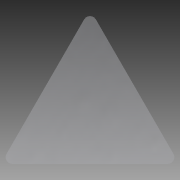
# Autodesk Inventor part: g16-pixel
Saved by Autodesk Inventor 2013 (Build 170138000, 138)
## iProperties
Created: 2013-03-21
Part Number: g16-pixel
Material: Acrylic, Clear
Document SubType Name: Modeling
Designer: TechShop Member
Density: 1 g/cm^3
Author: TechShop Member
Autodesk Inventor part; units mm, degrees
ref_plane "YZ Plane" through (0, 0, 0) normal (1, 0, 0) x (0, 1, 0)
ref_plane "XZ Plane" through (0, 0, 0) normal (0, 1, 0) x (-1, 0, 0)
ref_plane "XY Plane" through (0, 0, 0) normal (0, 0, 1) x (1, 0, 0)
sketch "Sketch1" plane through (0, 0, 0) normal (0, 1, 0) x (-1, 0, 0)
  line L0 (33.333, 0) -> (0, 0) construction
  line L1 (0, 0) -> (16.6665, 28.8672) construction
  line L2 (16.6665, 28.8672) -> (33.333, 0) construction
  line L3 (32.467, 0.5) -> (0.866, 0.5) construction
  line L4 (0.866, 0.5) -> (16.6665, 27.8672) construction
  line L5 (16.6665, 27.8672) -> (32.467, 0.5) construction
  line L6 (16.6665, 0.5) -> (16.6665, 0) construction
  line L7 (8.7663, 14.1836) -> (8.3333, 14.4336) construction
  line L8 (24.5667, 14.1836) -> (24.9998, 14.4336) construction
  arc A0 (1.9053, 2.3) -> (2.9445, 0.5) centre (2.9445, 1.7) ccw projected
  arc A1 (17.7057, 26.0672) -> (15.6273, 26.0672) centre (16.6665, 25.4672) ccw projected
  arc A2 (30.3885, 0.5) -> (31.4277, 2.3) centre (30.3885, 1.7) ccw projected
  line L9 (30.3885, 0.5) -> (2.9445, 0.5) projected
  line L10 (1.9053, 2.3) -> (15.6273, 26.0672) projected
  line L11 (17.7057, 26.0672) -> (31.4277, 2.3) projected
  circle A3 centre (31.7742, 0.9) radius 0.4 construction
  line L12 (31.4277, 1.1) -> (32.1206, 0.7) construction
  circle A4 centre (33.333, 0) radius 3 construction
  line L13 (16.6665, 0) -> (16.6665, -0.5) construction
  line L14 (31.4277, 1.1) -> (30.7349, 1.5) construction
  point P0 (0, 0)
  constraints: 1 other
extrude "Extrusion1" add sketch "Sketch1" along normal blind 2.75
sketch "Triangle Hole Template" plane through (0, 0, 0) normal (0, 0, 1) x (1, 0, 0)
  line L0 (-99.9974, -57.7156) -> (-66.6644, -57.7156) construction
  line L1 (-66.6644, -57.7156) -> (-83.3309, -86.5829) construction
  line L2 (-83.3309, -86.5829) -> (-99.9974, -57.7156) construction
  line L3 (-99.1314, -58.2156) -> (-67.5304, -58.2156) construction
  line L4 (-67.5304, -58.2156) -> (-83.3309, -85.5829) construction
  line L5 (-83.3309, -85.5829) -> (-99.1314, -58.2156) construction
  line L6 (-83.3309, -58.2156) -> (-83.3309, -57.7156) construction
  line L7 (-75.4307, -71.8992) -> (-74.9976, -72.1492) construction
  line L8 (-91.2311, -71.8992) -> (-91.6641, -72.1492) construction
  arc A0 (-68.5696, -60.0156) -> (-69.6089, -58.2156) centre (-69.6089, -59.4156) ccw
  arc A1 (-84.3701, -83.7829) -> (-82.2917, -83.7829) centre (-83.3309, -83.1829) ccw
  arc A2 (-97.0529, -58.2156) -> (-98.0921, -60.0156) centre (-97.0529, -59.4156) ccw
  line L9 (-97.0529, -58.2156) -> (-69.6089, -58.2156)
  line L10 (-68.5696, -60.0156) -> (-82.2917, -83.7829)
  line L11 (-84.3701, -83.7829) -> (-98.0921, -60.0156)
  circle A3 centre (-98.4385, -58.6156) radius 0.4 construction
  line L12 (-98.0921, -58.8156) -> (-98.785, -58.4156) construction
  circle A4 centre (-99.9974, -57.7156) radius 3 construction
  line L13 (-83.3309, -57.7156) -> (-83.3309, -57.2156) construction
  line L14 (-98.0921, -58.8156) -> (-97.3993, -59.2156) construction
  point P0 (-85.6081, -66.0431)
  dimension "d24" = 6
  dimension "Pixel_BorderWidth" = 1
  dimension "Pixel_Stride" = 33.333
  measures "Pixel_BorderWidth" distance of L13.end L6.start
  measures "Pixel_Stride" distance of L0.start L0.end
sketch "Triangle Hole Template x16" plane through (0, 0, 0) normal (0, 0, 1) x (1, 0, 0)
  line L0 (-16.6681, -28.8484) -> (-50.0011, -28.8484) construction
  line L1 (-50.0011, -28.8484) -> (-33.3346, 0.0188) construction
  line L2 (-33.3346, 0.0188) -> (-16.6681, -28.8484) construction
  line L3 (-17.5341, -28.3484) -> (-49.1351, -28.3484) construction
  line L4 (-49.1351, -28.3484) -> (-33.3346, -0.9812) construction
  line L5 (-33.3346, -0.9812) -> (-17.5341, -28.3484) construction
  line L6 (-33.3346, -28.3484) -> (-33.3346, -28.8484) construction
  line L7 (-41.2348, -14.6648) -> (-41.6679, -14.4148) construction
  line L8 (-25.4344, -14.6648) -> (-25.0014, -14.4148) construction
  arc A0 (-48.0959, -26.5484) -> (-47.0566, -28.3484) centre (-47.0566, -27.1484) ccw
  arc A1 (-32.2954, -2.7812) -> (-34.3738, -2.7812) centre (-33.3346, -3.3812) ccw
  arc A2 (-19.6126, -28.3484) -> (-18.5734, -26.5484) centre (-19.6126, -27.1484) ccw
  line L9 (-19.6126, -28.3484) -> (-47.0566, -28.3484)
  line L10 (-48.0959, -26.5484) -> (-34.3738, -2.7812)
  line L11 (-32.2954, -2.7812) -> (-18.5734, -26.5484)
  circle A3 centre (-18.227, -27.9484) radius 0.4 construction
  line L12 (-18.5734, -27.7484) -> (-17.8805, -28.1484) construction
  circle A4 centre (-16.6681, -28.8484) radius 3 construction
  line L13 (-33.3346, -28.8484) -> (-33.3346, -29.3484) construction
  line L14 (-18.5734, -27.7484) -> (-19.2662, -27.3484) construction
  line L15 (-49.9979, -28.8484) -> (-16.6649, -28.8484) construction
  line L16 (-16.6649, -28.8484) -> (-33.3314, -57.7156) construction
  line L17 (-33.3314, -57.7156) -> (-49.9979, -28.8484) construction
  line L18 (-49.1319, -29.3484) -> (-17.5309, -29.3484) construction
  line L19 (-17.5309, -29.3484) -> (-33.3314, -56.7156) construction
  line L20 (-33.3314, -56.7156) -> (-49.1319, -29.3484) construction
  line L21 (-33.3314, -29.3484) -> (-33.3314, -28.8484) construction
  line L22 (-25.4312, -43.032) -> (-24.9981, -43.282) construction
  line L23 (-41.2316, -43.032) -> (-41.6646, -43.282) construction
  arc A5 (-18.5701, -31.1484) -> (-19.6094, -29.3484) centre (-19.6094, -30.5484) ccw
  arc A6 (-34.3706, -54.9156) -> (-32.2922, -54.9156) centre (-33.3314, -54.3156) ccw
  arc A7 (-47.0534, -29.3484) -> (-48.0926, -31.1484) centre (-47.0534, -30.5484) ccw
  line L24 (-47.0534, -29.3484) -> (-19.6094, -29.3484)
  line L25 (-18.5701, -31.1484) -> (-32.2922, -54.9156)
  line L26 (-34.3706, -54.9156) -> (-48.0926, -31.1484)
  circle A8 centre (-48.439, -29.7484) radius 0.4 construction
  line L27 (-48.0926, -29.9484) -> (-48.7855, -29.5484) construction
  circle A9 centre (-49.9979, -28.8484) radius 3 construction
  line L28 (-33.3314, -28.8484) -> (-33.3314, -28.3484) construction
  line L29 (-48.0926, -29.9484) -> (-47.3998, -30.3484) construction
  line L30 (-66.6676, 0.0188) -> (-33.3346, 0.0188) construction
  line L31 (-33.3346, 0.0188) -> (-50.0011, -28.8484) construction
  line L32 (-50.0011, -28.8484) -> (-66.6676, 0.0188) construction
  line L33 (-65.8016, -0.4812) -> (-34.2006, -0.4812) construction
  line L34 (-34.2006, -0.4812) -> (-50.0011, -27.8484) construction
  line L35 (-50.0011, -27.8484) -> (-65.8016, -0.4812) construction
  line L36 (-50.0011, -0.4812) -> (-50.0011, 0.0188) construction
  line L37 (-42.1009, -14.1648) -> (-41.6679, -14.4148) construction
  line L38 (-57.9013, -14.1648) -> (-58.3344, -14.4148) construction
  arc A10 (-35.2399, -2.2812) -> (-36.2791, -0.4812) centre (-36.2791, -1.6812) ccw
  arc A11 (-51.0403, -26.0484) -> (-48.9619, -26.0484) centre (-50.0011, -25.4484) ccw
  arc A12 (-63.7231, -0.4812) -> (-64.7624, -2.2812) centre (-63.7231, -1.6812) ccw
  line L39 (-63.7231, -0.4812) -> (-36.2791, -0.4812)
  line L40 (-35.2399, -2.2812) -> (-48.9619, -26.0484)
  line L41 (-51.0403, -26.0484) -> (-64.7624, -2.2812)
  circle A13 centre (-65.1088, -0.8812) radius 0.4 construction
  line L42 (-64.7624, -1.0812) -> (-65.4552, -0.6812) construction
  circle A14 centre (-66.6676, 0.0188) radius 3 construction
  line L43 (-50.0011, 0.0188) -> (-50.0011, 0.5188) construction
  line L44 (-64.7624, -1.0812) -> (-64.0695, -1.4812) construction
  line L45 (-33.3314, 0.0188) -> (0.0016, 0.0188) construction
  line L46 (0.0016, 0.0188) -> (-16.6649, -28.8484) construction
  line L47 (-16.6649, -28.8484) -> (-33.3314, 0.0188) construction
  line L48 (-32.4654, -0.4812) -> (-0.8644, -0.4812) construction
  line L49 (-0.8644, -0.4812) -> (-16.6649, -27.8484) construction
  line L50 (-16.6649, -27.8484) -> (-32.4654, -0.4812) construction
  line L51 (-16.6649, -0.4812) -> (-16.6649, 0.0188) construction
  line L52 (-8.7647, -14.1648) -> (-8.3316, -14.4148) construction
  line L53 (-24.5651, -14.1648) -> (-24.9981, -14.4148) construction
  arc A15 (-1.9036, -2.2812) -> (-2.9429, -0.4812) centre (-2.9429, -1.6812) ccw
  arc A16 (-17.7041, -26.0484) -> (-15.6257, -26.0484) centre (-16.6649, -25.4484) ccw
  arc A17 (-30.3869, -0.4812) -> (-31.4261, -2.2812) centre (-30.3869, -1.6812) ccw
  line L54 (-30.3869, -0.4812) -> (-2.9429, -0.4812)
  line L55 (-1.9036, -2.2812) -> (-15.6257, -26.0484)
  line L56 (-17.7041, -26.0484) -> (-31.4261, -2.2812)
  circle A18 centre (-31.7725, -0.8812) radius 0.4 construction
  line L57 (-31.4261, -1.0812) -> (-32.119, -0.6812) construction
  circle A19 centre (-33.3314, 0.0188) radius 3 construction
  line L58 (-16.6649, 0.0188) -> (-16.6649, 0.5188) construction
  line L59 (-31.4261, -1.0812) -> (-30.7333, -1.4812) construction
  line L60 (-83.317, -28.8188) -> (-49.984, -28.8188) construction
  line L61 (-49.984, -28.8188) -> (-66.6505, -57.686) construction
  line L62 (-66.6505, -57.686) -> (-83.317, -28.8188) construction
  line L63 (-82.451, -29.3188) -> (-50.85, -29.3188) construction
  line L64 (-50.85, -29.3188) -> (-66.6505, -56.686) construction
  line L65 (-66.6505, -56.686) -> (-82.451, -29.3188) construction
  line L66 (-66.6505, -29.3188) -> (-66.6505, -28.8188) construction
  line L67 (-58.7503, -43.0024) -> (-58.3173, -43.2524) construction
  line L68 (-74.5507, -43.0024) -> (-74.9838, -43.2524) construction
  arc A20 (-51.8893, -31.1188) -> (-52.9285, -29.3188) centre (-52.9285, -30.5188) ccw
  arc A21 (-67.6897, -54.886) -> (-65.6113, -54.886) centre (-66.6505, -54.286) ccw
  arc A22 (-80.3725, -29.3188) -> (-81.4117, -31.1188) centre (-80.3725, -30.5188) ccw
  line L69 (-80.3725, -29.3188) -> (-52.9285, -29.3188)
  line L70 (-51.8893, -31.1188) -> (-65.6113, -54.886)
  line L71 (-67.6897, -54.886) -> (-81.4117, -31.1188)
  circle A23 centre (-81.7582, -29.7188) radius 0.4 construction
  line L72 (-81.4117, -29.9188) -> (-82.1046, -29.5188) construction
  circle A24 centre (-83.317, -28.8188) radius 3 construction
  line L73 (-66.6505, -28.8188) -> (-66.6505, -28.3188) construction
  line L74 (-81.4117, -29.9188) -> (-80.7189, -30.3188) construction
  line L75 (-99.9974, 0.0188) -> (-66.6644, 0.0188) construction
  line L76 (-66.6644, 0.0188) -> (-83.3309, -28.8484) construction
  line L77 (-83.3309, -28.8484) -> (-99.9974, 0.0188) construction
  line L78 (-99.1314, -0.4812) -> (-67.5304, -0.4812) construction
  line L79 (-67.5304, -0.4812) -> (-83.3309, -27.8484) construction
  line L80 (-83.3309, -27.8484) -> (-99.1314, -0.4812) construction
  line L81 (-83.3309, -0.4812) -> (-83.3309, 0.0188) construction
  line L82 (-75.4307, -14.1648) -> (-74.9976, -14.4148) construction
  line L83 (-91.2311, -14.1648) -> (-91.6641, -14.4148) construction
  arc A25 (-68.5696, -2.2812) -> (-69.6089, -0.4812) centre (-69.6089, -1.6812) ccw
  arc A26 (-84.3701, -26.0484) -> (-82.2917, -26.0484) centre (-83.3309, -25.4484) ccw
  arc A27 (-97.0529, -0.4812) -> (-98.0921, -2.2812) centre (-97.0529, -1.6812) ccw
  line L84 (-97.0529, -0.4812) -> (-69.6089, -0.4812)
  line L85 (-68.5696, -2.2812) -> (-82.2917, -26.0484)
  line L86 (-84.3701, -26.0484) -> (-98.0921, -2.2812)
  circle A28 centre (-98.4385, -0.8812) radius 0.4 construction
  line L87 (-98.0921, -1.0812) -> (-98.785, -0.6812) construction
  circle A29 centre (-99.9974, 0.0188) radius 3 construction
  line L88 (-83.3309, 0.0188) -> (-83.3309, 0.5188) construction
  line L89 (-98.0921, -1.0812) -> (-97.3993, -1.4812) construction
  line L90 (-133.3304, -0.008) -> (-99.9974, -0.008) construction
  line L91 (-99.9974, -0.008) -> (-116.6639, -28.8752) construction
  line L92 (-116.6639, -28.8752) -> (-133.3304, -0.008) construction
  line L93 (-132.4644, -0.508) -> (-100.8634, -0.508) construction
  line L94 (-100.8634, -0.508) -> (-116.6639, -27.8752) construction
  line L95 (-116.6639, -27.8752) -> (-132.4644, -0.508) construction
  line L96 (-116.6639, -0.508) -> (-116.6639, -0.008) construction
  line L97 (-108.7637, -14.1916) -> (-108.3306, -14.4416) construction
  line L98 (-124.5641, -14.1916) -> (-124.9971, -14.4416) construction
  arc A30 (-101.9026, -2.308) -> (-102.9419, -0.508) centre (-102.9419, -1.708) ccw
  arc A31 (-117.7031, -26.0752) -> (-115.6247, -26.0752) centre (-116.6639, -25.4752) ccw
  arc A32 (-130.3859, -0.508) -> (-131.4251, -2.308) centre (-130.3859, -1.708) ccw
  line L99 (-130.3859, -0.508) -> (-102.9419, -0.508)
  line L100 (-101.9026, -2.308) -> (-115.6247, -26.0752)
  line L101 (-117.7031, -26.0752) -> (-131.4251, -2.308)
  circle A33 centre (-131.7715, -0.908) radius 0.4 construction
  line L102 (-131.4251, -1.108) -> (-132.118, -0.708) construction
  circle A34 centre (-133.3304, -0.008) radius 3 construction
  line L103 (-116.6639, -0.008) -> (-116.6639, 0.492) construction
  line L104 (-131.4251, -1.108) -> (-130.7323, -1.508) construction
  line L105 (-116.6671, -28.8484) -> (-83.3341, -28.8484) construction
  line L106 (-83.3341, -28.8484) -> (-100.0006, -57.7156) construction
  line L107 (-100.0006, -57.7156) -> (-116.6671, -28.8484) construction
  line L108 (-115.8011, -29.3484) -> (-84.2001, -29.3484) construction
  line L109 (-84.2001, -29.3484) -> (-100.0006, -56.7156) construction
  line L110 (-100.0006, -56.7156) -> (-115.8011, -29.3484) construction
  line L111 (-100.0006, -29.3484) -> (-100.0006, -28.8484) construction
  line L112 (-92.1004, -43.032) -> (-91.6674, -43.282) construction
  line L113 (-107.9008, -43.032) -> (-108.3339, -43.282) construction
  arc A35 (-85.2394, -31.1484) -> (-86.2786, -29.3484) centre (-86.2786, -30.5484) ccw
  arc A36 (-101.0398, -54.9156) -> (-98.9614, -54.9156) centre (-100.0006, -54.3156) ccw
  arc A37 (-113.7226, -29.3484) -> (-114.7619, -31.1484) centre (-113.7226, -30.5484) ccw
  line L114 (-113.7226, -29.3484) -> (-86.2786, -29.3484)
  line L115 (-85.2394, -31.1484) -> (-98.9614, -54.9156)
  line L116 (-101.0398, -54.9156) -> (-114.7619, -31.1484)
  circle A38 centre (-115.1083, -29.7484) radius 0.4 construction
  line L117 (-114.7619, -29.9484) -> (-115.4547, -29.5484) construction
  circle A39 centre (-116.6671, -28.8484) radius 3 construction
  line L118 (-100.0006, -28.8484) -> (-100.0006, -28.3484) construction
  line L119 (-114.7619, -29.9484) -> (-114.069, -30.3484) construction
  line L120 (-99.9974, -57.7156) -> (-66.6644, -57.7156) construction
  line L121 (-66.6644, -57.7156) -> (-83.3309, -86.5829) construction
  line L122 (-83.3309, -86.5829) -> (-99.9974, -57.7156) construction
  line L123 (-99.1314, -58.2156) -> (-67.5304, -58.2156) construction
  line L124 (-67.5304, -58.2156) -> (-83.3309, -85.5829) construction
  line L125 (-83.3309, -85.5829) -> (-99.1314, -58.2156) construction
  line L126 (-83.3309, -58.2156) -> (-83.3309, -57.7156) construction
  line L127 (-75.4307, -71.8992) -> (-74.9976, -72.1492) construction
  line L128 (-91.2311, -71.8992) -> (-91.6641, -72.1492) construction
  arc A40 (-68.5696, -60.0156) -> (-69.6089, -58.2156) centre (-69.6089, -59.4156) ccw
  arc A41 (-84.3701, -83.7829) -> (-82.2917, -83.7829) centre (-83.3309, -83.1829) ccw
  arc A42 (-97.0529, -58.2156) -> (-98.0921, -60.0156) centre (-97.0529, -59.4156) ccw
  line L129 (-97.0529, -58.2156) -> (-69.6089, -58.2156)
  line L130 (-68.5696, -60.0156) -> (-82.2917, -83.7829)
  line L131 (-84.3701, -83.7829) -> (-98.0921, -60.0156)
  circle A43 centre (-98.4385, -58.6156) radius 0.4 construction
  line L132 (-98.0921, -58.8156) -> (-98.785, -58.4156) construction
  circle A44 centre (-99.9974, -57.7156) radius 3 construction
  line L133 (-83.3309, -57.7156) -> (-83.3309, -57.2156) construction
  line L134 (-98.0921, -58.8156) -> (-97.3993, -59.2156) construction
  line L135 (-83.3309, -86.5829) -> (-49.9979, -86.5829) construction
  line L136 (-49.9979, -86.5829) -> (-66.6644, -115.4501) construction
  line L137 (-66.6644, -115.4501) -> (-83.3309, -86.5829) construction
  line L138 (-82.4649, -87.0829) -> (-50.8639, -87.0829) construction
  line L139 (-50.8639, -87.0829) -> (-66.6644, -114.4501) construction
  line L140 (-66.6644, -114.4501) -> (-82.4649, -87.0829) construction
  line L141 (-66.6644, -87.0829) -> (-66.6644, -86.5829) construction
  line L142 (-58.7642, -100.7665) -> (-58.3311, -101.0165) construction
  line L143 (-74.5646, -100.7665) -> (-74.9976, -101.0165) construction
  arc A45 (-51.9031, -88.8829) -> (-52.9424, -87.0829) centre (-52.9424, -88.2829) ccw
  arc A46 (-67.7036, -112.6501) -> (-65.6252, -112.6501) centre (-66.6644, -112.0501) ccw
  arc A47 (-80.3864, -87.0829) -> (-81.4256, -88.8829) centre (-80.3864, -88.2829) ccw
  line L144 (-80.3864, -87.0829) -> (-52.9424, -87.0829)
  line L145 (-51.9031, -88.8829) -> (-65.6252, -112.6501)
  line L146 (-67.7036, -112.6501) -> (-81.4256, -88.8829)
  circle A48 centre (-81.772, -87.4829) radius 0.4 construction
  line L147 (-81.4256, -87.6829) -> (-82.1185, -87.2829) construction
  circle A49 centre (-83.3309, -86.5829) radius 3 construction
  line L148 (-66.6644, -86.5829) -> (-66.6644, -86.0829) construction
  line L149 (-81.4256, -87.6829) -> (-80.7328, -88.0829) construction
  line L150 (-66.6676, -57.7533) -> (-33.3346, -57.7533) construction
  line L151 (-33.3346, -57.7533) -> (-50.0011, -86.6205) construction
  line L152 (-50.0011, -86.6205) -> (-66.6676, -57.7533) construction
  line L153 (-65.8016, -58.2533) -> (-34.2006, -58.2533) construction
  line L154 (-34.2006, -58.2533) -> (-50.0011, -85.6205) construction
  line L155 (-50.0011, -85.6205) -> (-65.8016, -58.2533) construction
  line L156 (-50.0011, -58.2533) -> (-50.0011, -57.7533) construction
  line L157 (-42.1009, -71.9369) -> (-41.6679, -72.1869) construction
  line L158 (-57.9013, -71.9369) -> (-58.3344, -72.1869) construction
  arc A50 (-35.2399, -60.0533) -> (-36.2791, -58.2533) centre (-36.2791, -59.4533) ccw
  arc A51 (-51.0403, -83.8205) -> (-48.9619, -83.8205) centre (-50.0011, -83.2205) ccw
  arc A52 (-63.7231, -58.2533) -> (-64.7624, -60.0533) centre (-63.7231, -59.4533) ccw
  line L159 (-63.7231, -58.2533) -> (-36.2791, -58.2533)
  line L160 (-35.2399, -60.0533) -> (-48.9619, -83.8205)
  line L161 (-51.0403, -83.8205) -> (-64.7624, -60.0533)
  circle A53 centre (-65.1088, -58.6533) radius 0.4 construction
  line L162 (-64.7624, -58.8533) -> (-65.4552, -58.4533) construction
  circle A54 centre (-66.6676, -57.7533) radius 3 construction
  line L163 (-50.0011, -57.7533) -> (-50.0011, -57.2533) construction
  line L164 (-64.7624, -58.8533) -> (-64.0695, -59.2533) construction
  line L165 (-50.0011, -86.6205) -> (-83.3341, -86.6205) construction
  line L166 (-83.3341, -86.6205) -> (-66.6676, -57.7533) construction
  line L167 (-66.6676, -57.7533) -> (-50.0011, -86.6205) construction
  line L168 (-50.8671, -86.1205) -> (-82.4681, -86.1205) construction
  line L169 (-82.4681, -86.1205) -> (-66.6676, -58.7533) construction
  line L170 (-66.6676, -58.7533) -> (-50.8671, -86.1205) construction
  line L171 (-66.6676, -86.1205) -> (-66.6676, -86.6205) construction
  line L172 (-74.5678, -72.4369) -> (-75.0009, -72.1869) construction
  line L173 (-58.7674, -72.4369) -> (-58.3344, -72.1869) construction
  arc A55 (-81.4289, -84.3205) -> (-80.3896, -86.1205) centre (-80.3896, -84.9205) ccw
  arc A56 (-65.6284, -60.5533) -> (-67.7068, -60.5533) centre (-66.6676, -61.1533) ccw
  arc A57 (-52.9456, -86.1205) -> (-51.9064, -84.3205) centre (-52.9456, -84.9205) ccw
  line L174 (-52.9456, -86.1205) -> (-80.3896, -86.1205)
  line L175 (-81.4289, -84.3205) -> (-67.7068, -60.5533)
  line L176 (-65.6284, -60.5533) -> (-51.9064, -84.3205)
  circle A58 centre (-51.56, -85.7205) radius 0.4 construction
  line L177 (-51.9064, -85.5205) -> (-51.2135, -85.9205) construction
  circle A59 centre (-50.0011, -86.6205) radius 3 construction
  line L178 (-66.6676, -86.6205) -> (-66.6676, -87.1205) construction
  line L179 (-51.9064, -85.5205) -> (-52.5992, -85.1205) construction
  line L180 (-33.3346, -57.7533) -> (-66.6676, -57.7533) construction
  line L181 (-66.6676, -57.7533) -> (-50.0011, -28.886) construction
  line L182 (-50.0011, -28.886) -> (-33.3346, -57.7533) construction
  line L183 (-34.2006, -57.2533) -> (-65.8016, -57.2533) construction
  line L184 (-65.8016, -57.2533) -> (-50.0011, -29.886) construction
  line L185 (-50.0011, -29.886) -> (-34.2006, -57.2533) construction
  line L186 (-50.0011, -57.2533) -> (-50.0011, -57.7533) construction
  line L187 (-57.9013, -43.5697) -> (-58.3344, -43.3197) construction
  line L188 (-42.1009, -43.5697) -> (-41.6679, -43.3197) construction
  arc A60 (-64.7624, -55.4533) -> (-63.7231, -57.2533) centre (-63.7231, -56.0533) ccw
  arc A61 (-48.9619, -31.686) -> (-51.0403, -31.686) centre (-50.0011, -32.286) ccw
  arc A62 (-36.2791, -57.2533) -> (-35.2399, -55.4533) centre (-36.2791, -56.0533) ccw
  line L189 (-36.2791, -57.2533) -> (-63.7231, -57.2533)
  line L190 (-64.7624, -55.4533) -> (-51.0403, -31.686)
  line L191 (-48.9619, -31.686) -> (-35.2399, -55.4533)
  circle A63 centre (-34.8935, -56.8533) radius 0.4 construction
  line L192 (-35.2399, -56.6533) -> (-34.547, -57.0533) construction
  circle A64 centre (-33.3346, -57.7533) radius 3 construction
  line L193 (-50.0011, -57.7533) -> (-50.0011, -58.2533) construction
  line L194 (-35.2399, -56.6533) -> (-35.9327, -56.2533) construction
  line L195 (-66.6676, -57.7156) -> (-100.0006, -57.7156) construction
  line L196 (-100.0006, -57.7156) -> (-83.3341, -28.8484) construction
  line L197 (-83.3341, -28.8484) -> (-66.6676, -57.7156) construction
  line L198 (-67.5336, -57.2156) -> (-99.1346, -57.2156) construction
  line L199 (-99.1346, -57.2156) -> (-83.3341, -29.8484) construction
  line L200 (-83.3341, -29.8484) -> (-67.5336, -57.2156) construction
  line L201 (-83.3341, -57.2156) -> (-83.3341, -57.7156) construction
  line L202 (-91.2343, -43.532) -> (-91.6674, -43.282) construction
  line L203 (-75.4339, -43.532) -> (-75.0009, -43.282) construction
  arc A65 (-98.0954, -55.4156) -> (-97.0561, -57.2156) centre (-97.0561, -56.0156) ccw
  arc A66 (-82.2949, -31.6484) -> (-84.3733, -31.6484) centre (-83.3341, -32.2484) ccw
  arc A67 (-69.6121, -57.2156) -> (-68.5729, -55.4156) centre (-69.6121, -56.0156) ccw
  line L204 (-69.6121, -57.2156) -> (-97.0561, -57.2156)
  line L205 (-98.0954, -55.4156) -> (-84.3733, -31.6484)
  line L206 (-82.2949, -31.6484) -> (-68.5729, -55.4156)
  circle A68 centre (-68.2265, -56.8156) radius 0.4 construction
  line L207 (-68.5729, -56.6156) -> (-67.88, -57.0156) construction
  circle A69 centre (-66.6676, -57.7156) radius 3 construction
  line L208 (-83.3341, -57.7156) -> (-83.3341, -58.2156) construction
  line L209 (-68.5729, -56.6156) -> (-69.2657, -56.2156) construction
  line L210 (-83.3186, -28.8752) -> (-116.6516, -28.8752) construction
  line L211 (-116.6516, -28.8752) -> (-99.9851, -0.008) construction
  line L212 (-99.9851, -0.008) -> (-83.3186, -28.8752) construction
  line L213 (-84.1846, -28.3752) -> (-115.7856, -28.3752) construction
  line L214 (-115.7856, -28.3752) -> (-99.9851, -1.008) construction
  line L215 (-99.9851, -1.008) -> (-84.1846, -28.3752) construction
  line L216 (-99.9851, -28.3752) -> (-99.9851, -28.8752) construction
  line L217 (-107.8853, -14.6916) -> (-108.3184, -14.4416) construction
  line L218 (-92.0849, -14.6916) -> (-91.6519, -14.4416) construction
  arc A70 (-114.7464, -26.5752) -> (-113.7071, -28.3752) centre (-113.7071, -27.1752) ccw
  arc A71 (-98.9459, -2.808) -> (-101.0243, -2.808) centre (-99.9851, -3.408) ccw
  arc A72 (-86.2631, -28.3752) -> (-85.2239, -26.5752) centre (-86.2631, -27.1752) ccw
  line L219 (-86.2631, -28.3752) -> (-113.7071, -28.3752)
  line L220 (-114.7464, -26.5752) -> (-101.0243, -2.808)
  line L221 (-98.9459, -2.808) -> (-85.2239, -26.5752)
  circle A73 centre (-84.8775, -27.9752) radius 0.4 construction
  line L222 (-85.2239, -27.7752) -> (-84.531, -28.1752) construction
  circle A74 centre (-83.3186, -28.8752) radius 3 construction
  line L223 (-99.9851, -28.8752) -> (-99.9851, -29.3752) construction
  line L224 (-85.2239, -27.7752) -> (-85.9167, -27.3752) construction
  line L225 (-50.0011, -28.8484) -> (-83.3341, -28.8484) construction
  line L226 (-83.3341, -28.8484) -> (-66.6676, 0.0188) construction
  line L227 (-66.6676, 0.0188) -> (-50.0011, -28.8484) construction
  line L228 (-50.8671, -28.3484) -> (-82.4681, -28.3484) construction
  line L229 (-82.4681, -28.3484) -> (-66.6676, -0.9812) construction
  line L230 (-66.6676, -0.9812) -> (-50.8671, -28.3484) construction
  line L231 (-66.6676, -28.3484) -> (-66.6676, -28.8484) construction
  line L232 (-74.5678, -14.6648) -> (-75.0009, -14.4148) construction
  line L233 (-58.7674, -14.6648) -> (-58.3344, -14.4148) construction
  arc A75 (-81.4289, -26.5484) -> (-80.3896, -28.3484) centre (-80.3896, -27.1484) ccw
  arc A76 (-65.6284, -2.7812) -> (-67.7068, -2.7812) centre (-66.6676, -3.3812) ccw
  arc A77 (-52.9456, -28.3484) -> (-51.9064, -26.5484) centre (-52.9456, -27.1484) ccw
  line L234 (-52.9456, -28.3484) -> (-80.3896, -28.3484)
  line L235 (-81.4289, -26.5484) -> (-67.7068, -2.7812)
  line L236 (-65.6284, -2.7812) -> (-51.9064, -26.5484)
  circle A78 centre (-51.56, -27.9484) radius 0.4 construction
  line L237 (-51.9064, -27.7484) -> (-51.2135, -28.1484) construction
  circle A79 centre (-50.0011, -28.8484) radius 3 construction
  line L238 (-66.6676, -28.8484) -> (-66.6676, -29.3484) construction
  line L239 (-51.9064, -27.7484) -> (-52.5992, -27.3484) construction
  point P0 (-67.2349, -38.1612)
derived "g16-bezel.ipt"
equation "\"d1\" = LayerThickness"
equation "\"LayerThickness\" = 2.75"
body "Solid1"
